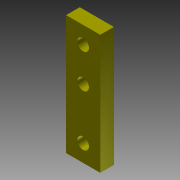
# Autodesk Inventor part: 13_0204_064
Saved by Autodesk Inventor 2012 SP1 (Build 160190100, 190)
## iProperties
Created: 2013-04-30
Part Number: 13_0204_064
Material: Default
Document SubType Name: Modeling
Designer: vogel
Density: 1 g/cm^3
Author: vogel
Autodesk Inventor part; units mm, degrees
ref_plane "YZ Plane" through (0, 0, 0) normal (1, 0, 0) x (0, 1, 0)
ref_plane "XZ Plane" through (0, 0, 0) normal (0, 1, 0) x (-1, 0, 0)
ref_plane "XY Plane" through (0, 0, 0) normal (0, 0, 1) x (1, 0, 0)
sketch "Skizze1" plane through (0, 0, 0) normal (0, 0, 1) x (1, 0, 0)
  line L0 (0, 0) -> (10, 0)
  line L1 (10, 0) -> (10, 4)
  line L2 (10, 4) -> (0, 4)
  line L3 (0, 4) -> (0, 0)
  dimension "d0" = 4
  dimension "d1" = 10
  constraints: 8 end point, 2 parallel, 1 horizontal, 1 perpendicular
  measures "d0" distance of L2.end L0.start
  measures "d1" distance of L0.start L0.end
extrude "Extrusion1" add sketch "Skizze1" along normal blind 40
sketch "Skizze2" plane through (0, 0, 0) normal (0, -1, 0) x (1, 0, 0)
  line L0 (0, 0) -> (10, 0) projected
  line L1 (10, 0) -> (10, 40) projected
  line L2 (10, 40) -> (0, 40) projected
  point P0 (5, 5)
  point P1 (5, 35)
  point P2 (5, 25)
  dimension "d4" = 5
  dimension "d5" = 5
  dimension "d13" = 5
  dimension "d14" = 10
  dimension "d15" = 5
  constraints: 1 vertical alignment
  measures "d4" distance from line of point (5, 5) L0
  measures "d5" distance from line of point (5, 5) L1
  measures "d13" distance from line of point (5, 35) L2
  measures "d14" distance of point (5, 25) point (5, 35)
  measures "d15" distance from line of point (5, 25) L1
hole "Bohrung2" at (5, 0, 5) at (5, 0, 35) at (5, 0, 25) direction (0, 1, 0) diameter 3.4 end through all
